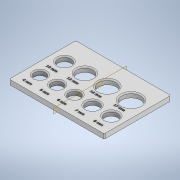
# Autodesk Inventor part: mmHexSocketSetOf9
Saved by Autodesk Inventor 2020.3 (Build 243373000, 373)
## iProperties
Created: 2020-03-13
Part Number: mmHexSocketSetOf9
Material: Generic
Document SubType Name: Modeling
Designer: robst
Density: 1 g/cm^3
Appearance: Default
Author: robst
Autodesk Inventor part; units mm, degrees
(part 1 of 2)
ref_plane "XZ Plane" through (0, 0, 0) normal (0, 1, 0) x (-1, 0, 0)
ref_plane "XY Plane" through (0, 0, 0) normal (0, 0, 1) x (1, 0, 0)
sketch "Sketch1" plane through (0, 0, 0) normal (0, 1, 0) x (-1, 0, 0)
  line L0 (63.5, 44.45) -> (-63.5, 44.45)
  line L1 (-63.5, 44.45) -> (-63.5, -44.45)
  line L2 (-63.5, -44.45) -> (63.5, -44.45)
  line L3 (63.5, -44.45) -> (63.5, 44.45)
  line L4 (63.5, 44.45) -> (-63.5, -44.45) construction
  line L5 (-63.5, 44.45) -> (63.5, -44.45) construction
  point P0 (0, 0)
  dimension "d3" = 88.9
  dimension "d13" = 127
  constraints: 12 end point, 2 midpoint, 2 parallel, 1 horizontal, 1 perpendicular
  measures "d3" distance of L2.end L0.start
  measures "d13" distance of L1.end L2.end
extrude "Extrusion1" add sketch "Sketch1" against normal blind 6.35
sketch "Sketch4" plane through (0, 0, 0) normal (0, 1, 0) x (1, 0, 0)
  line L0 (-63.5, -44.45) -> (-63.5, 44.45) construction
  line L1 (-63.5, -19.05) -> (63.5, -19.05) construction
  line L2 (63.5, 44.45) -> (63.5, -44.45) construction
  line L3 (-63.5, -44.45) -> (63.5, -44.45) projected
  circle A0 centre (-47.9975, -19.05) radius 7.62
  circle A1 centre (-24.8751, -19.05) radius 7.62
  circle A2 centre (-1.7526, -19.05) radius 7.62
  circle A3 centre (22.3859, -19.05) radius 8.636
  circle A4 centre (47.5403, -19.05) radius 8.636
  line L4 (-63.5, 12.7) -> (63.5, 12.7) construction
  circle A5 centre (-46.863, 12.7) radius 8.763
  circle A6 centre (-19.6215, 12.7) radius 10.6045
  circle A7 centre (10.414, 12.7) radius 11.557
  circle A8 centre (42.3545, 12.7) radius 12.5095
  point P0 (0, 0)
  dimension "d16" = 25.4
  dimension "hex4mmHole" = 15.24
  dimension "gap0" = 7.8825
  dimension "hex5mmHole" = 15.24
  dimension "gap1" = 23.1225
  dimension "hex6mmHole" = 15.24
  dimension "gap2" = 23.1225
  dimension "gap3" = 24.1385
  dimension "gap4" = 25.1545
  dimension "hex7mmHole" = 17.272
  dimension "hex8mmHole" = 17.272
  dimension "d27" = 7.3237
  dimension "frontToBackRowGap" = 31.75
  dimension "gap5" = 7.874
  dimension "hex10mmHole" = 17.526
  dimension "hex12mmHole" = 21.209
  dimension "gap6" = 27.2415
  dimension "hex14mmHole" = 23.114
  dimension "gap7" = 30.0355
  dimension "hex17mmHole" = 25.019
  dimension "gap8" = 31.9405
  dimension "d37" = 8.636
  constraints: 13 point on line, 9 centre point, 4 end point, 1 horizontal, 1 perpendicular
  measures "d16" distance between parallel lines of L1 L3
  measures "hex4mmHole" diameter of A0
  measures "gap0" distance edge to line of A0 L0
  measures "hex5mmHole" diameter of A1
  measures "gap1" distance of A1.centre A0.centre
  measures "hex6mmHole" diameter of A2
  measures "gap2" distance of A2.centre A1.centre
  measures "gap3" distance of A3.centre A2.centre
  measures "gap4" distance of A4.centre A3.centre
  measures "hex7mmHole" diameter of A3
  measures "hex8mmHole" diameter of A4
  measures "d27" distance edge to line of A4 L2
  measures "frontToBackRowGap" distance between parallel lines of L4 L1
  measures "gap5" distance edge to line of A5 L0
  measures "hex10mmHole" diameter of A5
  measures "hex12mmHole" diameter of A6
  measures "gap6" distance of A6.centre A5.centre
  measures "hex14mmHole" diameter of A7
  measures "gap7" distance of A7.centre A6.centre
  measures "hex17mmHole" diameter of A8
  measures "gap8" distance of A8.centre A7.centre
  measures "d37" distance edge to line of A8 L2
extrude "Extrusion3" cut sketch "Sketch4" against normal through all
sketch "Sketch7" plane through (0, 0, 0) normal (0, 1, 0) x (1, 0, 0)
  circle A0 centre (-47.9975, -19.05) radius 7.62 construction
  line L0 (63.5, -44.45) -> (-63.5, -44.45) construction
  line L1 (-55.6175, -35.6779) -> (-40.3775, -35.6779) construction
  line L2 (-32.4951, -35.6779) -> (-17.2551, -35.6779) construction
  line L3 (-9.3726, -35.6779) -> (5.8674, -35.6779) construction
  line L4 (13.7499, -35.6779) -> (30.7679, -35.6779) construction
  line L5 (38.6503, -35.6779) -> (55.6683, -35.6779) construction
  line L6 (-55.626, -3.81) -> (-38.354, -3.81) construction
  line L7 (-30.48, -3.81) -> (-7.62, -3.81) construction
  line L8 (0.254, -3.81) -> (23.114, -3.81) construction
  line L9 (30.988, -3.81) -> (55.626, -3.81) construction
  line L10 (-51.8572, -5.334) -> (-53.8702, -5.334)
  line L11 (-53.8702, -5.334) -> (-53.8702, -4.8029)
  line L12 (-53.8702, -4.8029) -> (-53.228, -4.8029)
  line L13 (-53.228, -4.8029) -> (-53.228, -3.19)
  line L14 (-53.228, -3.19) -> (-53.8702, -3.19)
  line L15 (-53.8702, -3.19) -> (-53.8702, -2.6936)
  spline S0 degree 2 poles (-53.8702, -2.6936) (-53.7294, -2.6936) (-53.4503, -2.6565) (-53.3663, -2.617) knots 0 0 0 1 2 2 2
  spline S1 degree 2 poles (-53.3663, -2.617) (-53.27, -2.5676) (-53.1613, -2.4021) (-53.1515, -2.2786) knots 0 0 0 1 2 2 2
  line L16 (-53.1515, -2.2786) -> (-52.4846, -2.2786)
  line L17 (-52.4846, -2.2786) -> (-52.4846, -4.8029)
  line L18 (-52.4846, -4.8029) -> (-51.8572, -4.8029)
  line L19 (-51.8572, -4.8029) -> (-51.8572, -5.334)
  spline S2 degree 2 poles (-49.0907, -3.81) (-49.0907, -4.2052) (-49.2167, -4.798) (-49.3575, -4.9981) knots 0 0 0 1 2 2 2
  spline S3 degree 2 poles (-49.3575, -4.9981) (-49.4958, -5.1957) (-49.9429, -5.3982) (-50.264, -5.3982) knots 0 0 0 1 2 2 2
  spline S4 degree 2 poles (-50.264, -5.3982) (-50.5876, -5.3982) (-51.0322, -5.1957) (-51.173, -4.9931) knots 0 0 0 1 2 2 2
  spline S5 degree 2 poles (-51.173, -4.9931) (-51.3138, -4.7931) (-51.4397, -4.2052) (-51.4397, -3.81) knots 0 0 0 1 2 2 2
  spline S6 degree 2 poles (-51.4397, -3.81) (-51.4397, -3.4049) (-51.3138, -2.8319) (-51.1705, -2.6244) knots 0 0 0 1 2 2 2
  spline S7 degree 2 poles (-51.1705, -2.6244) (-51.0272, -2.4219) (-50.5752, -2.2242) (-50.264, -2.2242) knots 0 0 0 1 2 2 2
  spline S8 degree 2 poles (-50.264, -2.2242) (-49.9355, -2.2242) (-49.4958, -2.4317) (-49.355, -2.6367) knots 0 0 0 1 2 2 2
  spline S9 degree 2 poles (-49.355, -2.6367) (-49.2167, -2.8368) (-49.0907, -3.4271) (-49.0907, -3.81) knots 0 0 0 1 2 2 2
  spline S10 degree 2 poles (-49.8589, -3.81) (-49.8589, -3.2444) (-50.0442, -2.7874) (-50.264, -2.7874) knots 0 0 0 1 2 2 2
  spline S11 degree 2 poles (-50.264, -2.7874) (-50.4838, -2.7874) (-50.6716, -3.2444) (-50.6716, -3.8125) knots 0 0 0 1 2 2 2
  spline S12 degree 2 poles (-50.6716, -3.8125) (-50.6716, -4.3707) (-50.4838, -4.8351) (-50.264, -4.8351) knots 0 0 0 1 2 2 2
  spline S13 degree 2 poles (-50.264, -4.8351) (-50.0466, -4.8351) (-49.8589, -4.3707) (-49.8589, -3.81) knots 0 0 0 1 2 2 2
  line L20 (-44.6842, -5.334) -> (-44.6842, -4.1854)
  spline S14 degree 2 poles (-44.6842, -4.1854) (-44.6842, -4.015) (-44.6966, -3.7828) (-44.7262, -3.7087) knots 0 0 0 1 2 2 2
  spline S15 degree 2 poles (-44.7262, -3.7087) (-44.7583, -3.6346) (-44.8868, -3.5679) (-45.0029, -3.5679) knots 0 0 0 1 2 2 2
  spline S16 degree 2 poles (-45.0029, -3.5679) (-45.0844, -3.5679) (-45.2425, -3.6396) (-45.3363, -3.7063) knots 0 0 0 1 2 2 2
  line L21 (-45.3363, -3.7063) -> (-45.3363, -5.334)
  line L22 (-45.3363, -5.334) -> (-46.0576, -5.334)
  line L23 (-46.0576, -5.334) -> (-46.0576, -4.1854)
  spline S17 degree 2 poles (-46.0576, -4.1854) (-46.0576, -4.0175) (-46.0724, -3.7828) (-46.102, -3.7087) knots 0 0 0 1 2 2 2
  spline S18 degree 2 poles (-46.102, -3.7087) (-46.1341, -3.6346) (-46.2626, -3.5679) (-46.3787, -3.5679) knots 0 0 0 1 2 2 2
  spline S19 degree 2 poles (-46.3787, -3.5679) (-46.4651, -3.5679) (-46.6356, -3.6494) (-46.7146, -3.7063) knots 0 0 0 1 2 2 2
  line L24 (-46.7146, -3.7063) -> (-46.7146, -5.334)
  line L25 (-46.7146, -5.334) -> (-47.4309, -5.334)
  line L26 (-47.4309, -5.334) -> (-47.4309, -3.0344)
  line L27 (-47.4309, -3.0344) -> (-46.7146, -3.0344)
  line L28 (-46.7146, -3.0344) -> (-46.7146, -3.2888)
  spline S20 degree 2 poles (-46.7146, -3.2888) (-46.5392, -3.1406) (-46.2255, -2.9727) (-46.0304, -2.9727) knots 0 0 0 1 2 2 2
  spline S21 degree 2 poles (-46.0304, -2.9727) (-45.8204, -2.9727) (-45.4993, -3.1727) (-45.4154, -3.3728) knots 0 0 0 1 2 2 2
  spline S22 degree 2 poles (-45.4154, -3.3728) (-45.2104, -3.1801) (-44.8448, -2.9727) (-44.6571, -2.9727) knots 0 0 0 1 2 2 2
  spline S23 degree 2 poles (-44.6571, -2.9727) (-44.4965, -2.9727) (-44.2421, -3.0739) (-44.1557, -3.1777) knots 0 0 0 1 2 2 2
  spline S24 degree 2 poles (-44.1557, -3.1777) (-44.0593, -3.2888) (-43.963, -3.5926) (-43.963, -3.8372) knots 0 0 0 1 2 2 2
  line L29 (-43.963, -3.8372) -> (-43.963, -5.334)
  line L30 (-43.963, -5.334) -> (-44.6842, -5.334)
  line L31 (-40.6878, -5.334) -> (-40.6878, -4.1854)
  spline S25 degree 2 poles (-40.6878, -4.1854) (-40.6878, -4.015) (-40.7001, -3.7828) (-40.7297, -3.7087) knots 0 0 0 1 2 2 2
  spline S26 degree 2 poles (-40.7297, -3.7087) (-40.7619, -3.6346) (-40.8903, -3.5679) (-41.0064, -3.5679) knots 0 0 0 1 2 2 2
  spline S27 degree 2 poles (-41.0064, -3.5679) (-41.0879, -3.5679) (-41.246, -3.6396) (-41.3398, -3.7063) knots 0 0 0 1 2 2 2
  line L32 (-41.3398, -3.7063) -> (-41.3398, -5.334)
  line L33 (-41.3398, -5.334) -> (-42.0611, -5.334)
  line L34 (-42.0611, -5.334) -> (-42.0611, -4.1854)
  spline S28 degree 2 poles (-42.0611, -4.1854) (-42.0611, -4.0175) (-42.0759, -3.7828) (-42.1055, -3.7087) knots 0 0 0 1 2 2 2
  spline S29 degree 2 poles (-42.1055, -3.7087) (-42.1377, -3.6346) (-42.2661, -3.5679) (-42.3822, -3.5679) knots 0 0 0 1 2 2 2
  spline S30 degree 2 poles (-42.3822, -3.5679) (-42.4686, -3.5679) (-42.6391, -3.6494) (-42.7181, -3.7063) knots 0 0 0 1 2 2 2
  line L35 (-42.7181, -3.7063) -> (-42.7181, -5.334)
  line L36 (-42.7181, -5.334) -> (-43.4344, -5.334)
  line L37 (-43.4344, -5.334) -> (-43.4344, -3.0344)
  line L38 (-43.4344, -3.0344) -> (-42.7181, -3.0344)
  line L39 (-42.7181, -3.0344) -> (-42.7181, -3.2888)
  spline S31 degree 2 poles (-42.7181, -3.2888) (-42.5427, -3.1406) (-42.229, -2.9727) (-42.0339, -2.9727) knots 0 0 0 1 2 2 2
  spline S32 degree 2 poles (-42.0339, -2.9727) (-41.824, -2.9727) (-41.5029, -3.1727) (-41.4189, -3.3728) knots 0 0 0 1 2 2 2
  spline S33 degree 2 poles (-41.4189, -3.3728) (-41.2139, -3.1801) (-40.8483, -2.9727) (-40.6606, -2.9727) knots 0 0 0 1 2 2 2
  spline S34 degree 2 poles (-40.6606, -2.9727) (-40.5, -2.9727) (-40.2456, -3.0739) (-40.1592, -3.1777) knots 0 0 0 1 2 2 2
  spline S35 degree 2 poles (-40.1592, -3.1777) (-40.0628, -3.2888) (-39.9665, -3.5926) (-39.9665, -3.8372) knots 0 0 0 1 2 2 2
  line L40 (-39.9665, -3.8372) -> (-39.9665, -5.334)
  line L41 (-39.9665, -5.334) -> (-40.6878, -5.334)
  line L42 (-23.9172, -5.334) -> (-25.9302, -5.334)
  line L43 (-25.9302, -5.334) -> (-25.9302, -4.8029)
  line L44 (-25.9302, -4.8029) -> (-25.288, -4.8029)
  line L45 (-25.288, -4.8029) -> (-25.288, -3.19)
  line L46 (-25.288, -3.19) -> (-25.9302, -3.19)
  line L47 (-25.9302, -3.19) -> (-25.9302, -2.6936)
  spline S36 degree 2 poles (-25.9302, -2.6936) (-25.7894, -2.6936) (-25.5103, -2.6565) (-25.4263, -2.617) knots 0 0 0 1 2 2 2
  spline S37 degree 2 poles (-25.4263, -2.617) (-25.33, -2.5676) (-25.2213, -2.4021) (-25.2115, -2.2786) knots 0 0 0 1 2 2 2
  line L48 (-25.2115, -2.2786) -> (-24.5446, -2.2786)
  line L49 (-24.5446, -2.2786) -> (-24.5446, -4.8029)
  line L50 (-24.5446, -4.8029) -> (-23.9172, -4.8029)
  line L51 (-23.9172, -4.8029) -> (-23.9172, -5.334)
  line L52 (-21.1112, -5.334) -> (-23.3515, -5.334)
  line L53 (-23.3515, -5.334) -> (-23.3515, -4.8375)
  spline S38 degree 2 poles (-23.3515, -4.8375) (-23.0675, -4.6103) (-22.613, -4.2101) (-22.4426, -4.0298) knots 0 0 0 1 2 2 2
  spline S39 degree 2 poles (-22.4426, -4.0298) (-22.2178, -3.7952) (-22.0177, -3.437) (-22.0177, -3.2493) knots 0 0 0 1 2 2 2
  spline S40 degree 2 poles (-22.0177, -3.2493) (-22.0177, -3.0369) (-22.2721, -2.8096) (-22.4994, -2.8096) knots 0 0 0 1 2 2 2
  spline S41 degree 2 poles (-22.4994, -2.8096) (-22.6155, -2.8096) (-22.8229, -2.8665) (-22.9292, -2.9109) knots 0 0 0 1 2 2 2
  spline S42 degree 2 poles (-22.9292, -2.9109) (-23.0329, -2.9578) (-23.1811, -3.0566) (-23.2182, -3.0813) knots 0 0 0 1 2 2 2
  line L54 (-23.2182, -3.0813) -> (-23.2774, -3.0813)
  line L55 (-23.2774, -3.0813) -> (-23.2774, -2.4169)
  spline S43 degree 2 poles (-23.2774, -2.4169) (-23.149, -2.3552) (-22.6006, -2.2267) (-22.3462, -2.2267) knots 0 0 0 1 2 2 2
  spline S44 degree 2 poles (-22.3462, -2.2267) (-21.8028, -2.2267) (-21.2446, -2.7108) (-21.2446, -3.148) knots 0 0 0 1 2 2 2
  spline S45 degree 2 poles (-21.2446, -3.148) (-21.2446, -3.4173) (-21.499, -3.936) (-21.793, -4.2324) knots 0 0 0 1 2 2 2
  spline S46 degree 2 poles (-21.793, -4.2324) (-21.9782, -4.4152) (-22.3265, -4.6992) (-22.403, -4.7585) knots 0 0 0 1 2 2 2
  line L56 (-22.403, -4.7585) -> (-21.1112, -4.7585)
  line L57 (-21.1112, -4.7585) -> (-21.1112, -5.334)
  line L58 (-16.7442, -5.334) -> (-16.7442, -4.1854)
  spline S47 degree 2 poles (-16.7442, -4.1854) (-16.7442, -4.015) (-16.7566, -3.7828) (-16.7862, -3.7087) knots 0 0 0 1 2 2 2
  spline S48 degree 2 poles (-16.7862, -3.7087) (-16.8183, -3.6346) (-16.9468, -3.5679) (-17.0629, -3.5679) knots 0 0 0 1 2 2 2
  spline S49 degree 2 poles (-17.0629, -3.5679) (-17.1444, -3.5679) (-17.3025, -3.6396) (-17.3963, -3.7063) knots 0 0 0 1 2 2 2
  line L59 (-17.3963, -3.7063) -> (-17.3963, -5.334)
  line L60 (-17.3963, -5.334) -> (-18.1176, -5.334)
  line L61 (-18.1176, -5.334) -> (-18.1176, -4.1854)
  spline S50 degree 2 poles (-18.1176, -4.1854) (-18.1176, -4.0175) (-18.1324, -3.7828) (-18.162, -3.7087) knots 0 0 0 1 2 2 2
  spline S51 degree 2 poles (-18.162, -3.7087) (-18.1941, -3.6346) (-18.3226, -3.5679) (-18.4387, -3.5679) knots 0 0 0 1 2 2 2
  spline S52 degree 2 poles (-18.4387, -3.5679) (-18.5251, -3.5679) (-18.6956, -3.6494) (-18.7746, -3.7063) knots 0 0 0 1 2 2 2
  line L62 (-18.7746, -3.7063) -> (-18.7746, -5.334)
  line L63 (-18.7746, -5.334) -> (-19.4909, -5.334)
  line L64 (-19.4909, -5.334) -> (-19.4909, -3.0344)
  line L65 (-19.4909, -3.0344) -> (-18.7746, -3.0344)
  line L66 (-18.7746, -3.0344) -> (-18.7746, -3.2888)
  spline S53 degree 2 poles (-18.7746, -3.2888) (-18.5992, -3.1406) (-18.2855, -2.9727) (-18.0904, -2.9727) knots 0 0 0 1 2 2 2
  spline S54 degree 2 poles (-18.0904, -2.9727) (-17.8804, -2.9727) (-17.5593, -3.1727) (-17.4754, -3.3728) knots 0 0 0 1 2 2 2
  spline S55 degree 2 poles (-17.4754, -3.3728) (-17.2704, -3.1801) (-16.9048, -2.9727) (-16.7171, -2.9727) knots 0 0 0 1 2 2 2
  spline S56 degree 2 poles (-16.7171, -2.9727) (-16.5565, -2.9727) (-16.3021, -3.0739) (-16.2157, -3.1777) knots 0 0 0 1 2 2 2
  spline S57 degree 2 poles (-16.2157, -3.1777) (-16.1193, -3.2888) (-16.023, -3.5926) (-16.023, -3.8372) knots 0 0 0 1 2 2 2
  line L67 (-16.023, -3.8372) -> (-16.023, -5.334)
  line L68 (-16.023, -5.334) -> (-16.7442, -5.334)
  line L69 (-12.7478, -5.334) -> (-12.7478, -4.1854)
  spline S58 degree 2 poles (-12.7478, -4.1854) (-12.7478, -4.015) (-12.7601, -3.7828) (-12.7897, -3.7087) knots 0 0 0 1 2 2 2
  spline S59 degree 2 poles (-12.7897, -3.7087) (-12.8219, -3.6346) (-12.9503, -3.5679) (-13.0664, -3.5679) knots 0 0 0 1 2 2 2
  spline S60 degree 2 poles (-13.0664, -3.5679) (-13.1479, -3.5679) (-13.306, -3.6396) (-13.3998, -3.7063) knots 0 0 0 1 2 2 2
  line L70 (-13.3998, -3.7063) -> (-13.3998, -5.334)
  line L71 (-13.3998, -5.334) -> (-14.1211, -5.334)
  line L72 (-14.1211, -5.334) -> (-14.1211, -4.1854)
  spline S61 degree 2 poles (-14.1211, -4.1854) (-14.1211, -4.0175) (-14.1359, -3.7828) (-14.1655, -3.7087) knots 0 0 0 1 2 2 2
  spline S62 degree 2 poles (-14.1655, -3.7087) (-14.1977, -3.6346) (-14.3261, -3.5679) (-14.4422, -3.5679) knots 0 0 0 1 2 2 2
  spline S63 degree 2 poles (-14.4422, -3.5679) (-14.5286, -3.5679) (-14.6991, -3.6494) (-14.7781, -3.7063) knots 0 0 0 1 2 2 2
  line L73 (-14.7781, -3.7063) -> (-14.7781, -5.334)
  line L74 (-14.7781, -5.334) -> (-15.4944, -5.334)
  line L75 (-15.4944, -5.334) -> (-15.4944, -3.0344)
  line L76 (-15.4944, -3.0344) -> (-14.7781, -3.0344)
  line L77 (-14.7781, -3.0344) -> (-14.7781, -3.2888)
  spline S64 degree 2 poles (-14.7781, -3.2888) (-14.6027, -3.1406) (-14.289, -2.9727) (-14.0939, -2.9727) knots 0 0 0 1 2 2 2
  spline S65 degree 2 poles (-14.0939, -2.9727) (-13.884, -2.9727) (-13.5629, -3.1727) (-13.4789, -3.3728) knots 0 0 0 1 2 2 2
  spline S66 degree 2 poles (-13.4789, -3.3728) (-13.2739, -3.1801) (-12.9083, -2.9727) (-12.7206, -2.9727) knots 0 0 0 1 2 2 2
  spline S67 degree 2 poles (-12.7206, -2.9727) (-12.56, -2.9727) (-12.3056, -3.0739) (-12.2192, -3.1777) knots 0 0 0 1 2 2 2
  spline S68 degree 2 poles (-12.2192, -3.1777) (-12.1228, -3.2888) (-12.0265, -3.5926) (-12.0265, -3.8372) knots 0 0 0 1 2 2 2
  line L78 (-12.0265, -3.8372) -> (-12.0265, -5.334)
  line L79 (-12.0265, -5.334) -> (-12.7478, -5.334)
  line L80 (6.8168, -5.334) -> (4.8038, -5.334)
  line L81 (4.8038, -5.334) -> (4.8038, -4.8029)
  line L82 (4.8038, -4.8029) -> (5.446, -4.8029)
  line L83 (5.446, -4.8029) -> (5.446, -3.19)
  line L84 (5.446, -3.19) -> (4.8038, -3.19)
  line L85 (4.8038, -3.19) -> (4.8038, -2.6936)
  spline S69 degree 2 poles (4.8038, -2.6936) (4.9446, -2.6936) (5.2237, -2.6565) (5.3077, -2.617) knots 0 0 0 1 2 2 2
  spline S70 degree 2 poles (5.3077, -2.617) (5.404, -2.5676) (5.5127, -2.4021) (5.5225, -2.2786) knots 0 0 0 1 2 2 2
  line L86 (5.5225, -2.2786) -> (6.1894, -2.2786)
  line L87 (6.1894, -2.2786) -> (6.1894, -4.8029)
  line L88 (6.1894, -4.8029) -> (6.8168, -4.8029)
  line L89 (6.8168, -4.8029) -> (6.8168, -5.334)
  line L90 (9.6598, -4.6226) -> (9.2473, -4.6226)
  line L91 (9.2473, -4.6226) -> (9.2473, -5.3414)
  line L92 (9.2473, -5.3414) -> (8.5088, -5.3414)
  line L93 (8.5088, -5.3414) -> (8.5088, -4.6226)
  line L94 (8.5088, -4.6226) -> (7.1651, -4.6226)
  line L95 (7.1651, -4.6226) -> (7.1651, -4.0545)
  line L96 (7.1651, -4.0545) -> (8.4841, -2.286)
  line L97 (8.4841, -2.286) -> (9.2473, -2.286)
  line L98 (9.2473, -2.286) -> (9.2473, -4.0743)
  line L99 (9.2473, -4.0743) -> (9.6598, -4.0743)
  line L100 (9.6598, -4.0743) -> (9.6598, -4.6226)
  line L101 (8.5088, -4.0743) -> (8.5088, -3.0369)
  line L102 (8.5088, -3.0369) -> (7.7357, -4.0743)
  line L103 (7.7357, -4.0743) -> (8.5088, -4.0743)
  line L104 (13.9898, -5.334) -> (13.9898, -4.1854)
  spline S71 degree 2 poles (13.9898, -4.1854) (13.9898, -4.015) (13.9774, -3.7828) (13.9478, -3.7087) knots 0 0 0 1 2 2 2
  spline S72 degree 2 poles (13.9478, -3.7087) (13.9157, -3.6346) (13.7872, -3.5679) (13.6711, -3.5679) knots 0 0 0 1 2 2 2
  spline S73 degree 2 poles (13.6711, -3.5679) (13.5896, -3.5679) (13.4315, -3.6396) (13.3377, -3.7063) knots 0 0 0 1 2 2 2
  line L105 (13.3377, -3.7063) -> (13.3377, -5.334)
  line L106 (13.3377, -5.334) -> (12.6164, -5.334)
  line L107 (12.6164, -5.334) -> (12.6164, -4.1854)
  spline S74 degree 2 poles (12.6164, -4.1854) (12.6164, -4.0175) (12.6016, -3.7828) (12.572, -3.7087) knots 0 0 0 1 2 2 2
  spline S75 degree 2 poles (12.572, -3.7087) (12.5399, -3.6346) (12.4114, -3.5679) (12.2953, -3.5679) knots 0 0 0 1 2 2 2
  spline S76 degree 2 poles (12.2953, -3.5679) (12.2089, -3.5679) (12.0384, -3.6494) (11.9594, -3.7063) knots 0 0 0 1 2 2 2
  line L108 (11.9594, -3.7063) -> (11.9594, -5.334)
  line L109 (11.9594, -5.334) -> (11.2431, -5.334)
  line L110 (11.2431, -5.334) -> (11.2431, -3.0344)
  line L111 (11.2431, -3.0344) -> (11.9594, -3.0344)
  line L112 (11.9594, -3.0344) -> (11.9594, -3.2888)
  spline S77 degree 2 poles (11.9594, -3.2888) (12.1348, -3.1406) (12.4485, -2.9727) (12.6436, -2.9727) knots 0 0 0 1 2 2 2
  spline S78 degree 2 poles (12.6436, -2.9727) (12.8536, -2.9727) (13.1747, -3.1727) (13.2586, -3.3728) knots 0 0 0 1 2 2 2
  spline S79 degree 2 poles (13.2586, -3.3728) (13.4636, -3.1801) (13.8292, -2.9727) (14.0169, -2.9727) knots 0 0 0 1 2 2 2
  spline S80 degree 2 poles (14.0169, -2.9727) (14.1775, -2.9727) (14.4319, -3.0739) (14.5183, -3.1777) knots 0 0 0 1 2 2 2
  spline S81 degree 2 poles (14.5183, -3.1777) (14.6147, -3.2888) (14.711, -3.5926) (14.711, -3.8372) knots 0 0 0 1 2 2 2
  line L113 (14.711, -3.8372) -> (14.711, -5.334)
  line L114 (14.711, -5.334) -> (13.9898, -5.334)
  line L115 (17.9862, -5.334) -> (17.9862, -4.1854)
  spline S82 degree 2 poles (17.9862, -4.1854) (17.9862, -4.015) (17.9739, -3.7828) (17.9443, -3.7087) knots 0 0 0 1 2 2 2
  spline S83 degree 2 poles (17.9443, -3.7087) (17.9121, -3.6346) (17.7837, -3.5679) (17.6676, -3.5679) knots 0 0 0 1 2 2 2
  spline S84 degree 2 poles (17.6676, -3.5679) (17.5861, -3.5679) (17.428, -3.6396) (17.3342, -3.7063) knots 0 0 0 1 2 2 2
  line L116 (17.3342, -3.7063) -> (17.3342, -5.334)
  line L117 (17.3342, -5.334) -> (16.6129, -5.334)
  line L118 (16.6129, -5.334) -> (16.6129, -4.1854)
  spline S85 degree 2 poles (16.6129, -4.1854) (16.6129, -4.0175) (16.5981, -3.7828) (16.5685, -3.7087) knots 0 0 0 1 2 2 2
  spline S86 degree 2 poles (16.5685, -3.7087) (16.5363, -3.6346) (16.4079, -3.5679) (16.2918, -3.5679) knots 0 0 0 1 2 2 2
  spline S87 degree 2 poles (16.2918, -3.5679) (16.2054, -3.5679) (16.0349, -3.6494) (15.9559, -3.7063) knots 0 0 0 1 2 2 2
  line L119 (15.9559, -3.7063) -> (15.9559, -5.334)
  line L120 (15.9559, -5.334) -> (15.2396, -5.334)
  line L121 (15.2396, -5.334) -> (15.2396, -3.0344)
  line L122 (15.2396, -3.0344) -> (15.9559, -3.0344)
  line L123 (15.9559, -3.0344) -> (15.9559, -3.2888)
  spline S88 degree 2 poles (15.9559, -3.2888) (16.1313, -3.1406) (16.445, -2.9727) (16.6401, -2.9727) knots 0 0 0 1 2 2 2
  spline S89 degree 2 poles (16.6401, -2.9727) (16.85, -2.9727) (17.1711, -3.1727) (17.2551, -3.3728) knots 0 0 0 1 2 2 2
  spline S90 degree 2 poles (17.2551, -3.3728) (17.4601, -3.1801) (17.8257, -2.9727) (18.0134, -2.9727) knots 0 0 0 1 2 2 2
  spline S91 degree 2 poles (18.0134, -2.9727) (18.174, -2.9727) (18.4284, -3.0739) (18.5148, -3.1777) knots 0 0 0 1 2 2 2
  spline S92 degree 2 poles (18.5148, -3.1777) (18.6112, -3.2888) (18.7075, -3.5926) (18.7075, -3.8372) knots 0 0 0 1 2 2 2
  line L124 (18.7075, -3.8372) -> (18.7075, -5.334)
  line L125 (18.7075, -5.334) -> (17.9862, -5.334)
  line L126 (38.4398, -5.334) -> (36.4268, -5.334)
  line L127 (36.4268, -5.334) -> (36.4268, -4.8029)
  line L128 (36.4268, -4.8029) -> (37.069, -4.8029)
  line L129 (37.069, -4.8029) -> (37.069, -3.19)
  line L130 (37.069, -3.19) -> (36.4268, -3.19)
  line L131 (36.4268, -3.19) -> (36.4268, -2.6936)
  spline S93 degree 2 poles (36.4268, -2.6936) (36.5676, -2.6936) (36.8467, -2.6565) (36.9307, -2.617) knots 0 0 0 1 2 2 2
  spline S94 degree 2 poles (36.9307, -2.617) (37.027, -2.5676) (37.1357, -2.4021) (37.1455, -2.2786) knots 0 0 0 1 2 2 2
  line L132 (37.1455, -2.2786) -> (37.8124, -2.2786)
  line L133 (37.8124, -2.2786) -> (37.8124, -4.8029)
  line L134 (37.8124, -4.8029) -> (38.4398, -4.8029)
  line L135 (38.4398, -4.8029) -> (38.4398, -5.334)
  line L136 (41.1791, -2.8912) -> (39.8774, -5.334)
  line L137 (39.8774, -5.334) -> (39.0277, -5.334)
  line L138 (39.0277, -5.334) -> (40.3887, -2.8615)
  line L139 (40.3887, -2.8615) -> (38.9363, -2.8615)
  line L140 (38.9363, -2.8615) -> (38.9363, -2.286)
  line L141 (38.9363, -2.286) -> (41.1791, -2.286)
  line L142 (41.1791, -2.286) -> (41.1791, -2.8912)
  line L143 (45.6128, -5.334) -> (45.6128, -4.1854)
  spline S95 degree 2 poles (45.6128, -4.1854) (45.6128, -4.015) (45.6004, -3.7828) (45.5708, -3.7087) knots 0 0 0 1 2 2 2
  spline S96 degree 2 poles (45.5708, -3.7087) (45.5387, -3.6346) (45.4102, -3.5679) (45.2941, -3.5679) knots 0 0 0 1 2 2 2
  spline S97 degree 2 poles (45.2941, -3.5679) (45.2126, -3.5679) (45.0545, -3.6396) (44.9607, -3.7063) knots 0 0 0 1 2 2 2
  line L144 (44.9607, -3.7063) -> (44.9607, -5.334)
  line L145 (44.9607, -5.334) -> (44.2394, -5.334)
  line L146 (44.2394, -5.334) -> (44.2394, -4.1854)
  spline S98 degree 2 poles (44.2394, -4.1854) (44.2394, -4.0175) (44.2246, -3.7828) (44.195, -3.7087) knots 0 0 0 1 2 2 2
  spline S99 degree 2 poles (44.195, -3.7087) (44.1629, -3.6346) (44.0344, -3.5679) (43.9183, -3.5679) knots 0 0 0 1 2 2 2
  spline S100 degree 2 poles (43.9183, -3.5679) (43.8319, -3.5679) (43.6614, -3.6494) (43.5824, -3.7063) knots 0 0 0 1 2 2 2
  line L147 (43.5824, -3.7063) -> (43.5824, -5.334)
  line L148 (43.5824, -5.334) -> (42.8661, -5.334)
  line L149 (42.8661, -5.334) -> (42.8661, -3.0344)
  line L150 (42.8661, -3.0344) -> (43.5824, -3.0344)
  line L151 (43.5824, -3.0344) -> (43.5824, -3.2888)
  spline S101 degree 2 poles (43.5824, -3.2888) (43.7578, -3.1406) (44.0715, -2.9727) (44.2666, -2.9727) knots 0 0 0 1 2 2 2
  spline S102 degree 2 poles (44.2666, -2.9727) (44.4766, -2.9727) (44.7977, -3.1727) (44.8816, -3.3728) knots 0 0 0 1 2 2 2
  spline S103 degree 2 poles (44.8816, -3.3728) (45.0866, -3.1801) (45.4522, -2.9727) (45.6399, -2.9727) knots 0 0 0 1 2 2 2
  spline S104 degree 2 poles (45.6399, -2.9727) (45.8005, -2.9727) (46.0549, -3.0739) (46.1413, -3.1777) knots 0 0 0 1 2 2 2
  spline S105 degree 2 poles (46.1413, -3.1777) (46.2377, -3.2888) (46.334, -3.5926) (46.334, -3.8372) knots 0 0 0 1 2 2 2
  line L152 (46.334, -3.8372) -> (46.334, -5.334)
  line L153 (46.334, -5.334) -> (45.6128, -5.334)
  line L154 (49.6092, -5.334) -> (49.6092, -4.1854)
  spline S106 degree 2 poles (49.6092, -4.1854) (49.6092, -4.015) (49.5969, -3.7828) (49.5673, -3.7087) knots 0 0 0 1 2 2 2
  spline S107 degree 2 poles (49.5673, -3.7087) (49.5351, -3.6346) (49.4067, -3.5679) (49.2906, -3.5679) knots 0 0 0 1 2 2 2
  spline S108 degree 2 poles (49.2906, -3.5679) (49.2091, -3.5679) (49.051, -3.6396) (48.9572, -3.7063) knots 0 0 0 1 2 2 2
  line L155 (48.9572, -3.7063) -> (48.9572, -5.334)
  line L156 (48.9572, -5.334) -> (48.2359, -5.334)
  line L157 (48.2359, -5.334) -> (48.2359, -4.1854)
  spline S109 degree 2 poles (48.2359, -4.1854) (48.2359, -4.0175) (48.2211, -3.7828) (48.1915, -3.7087) knots 0 0 0 1 2 2 2
  spline S110 degree 2 poles (48.1915, -3.7087) (48.1593, -3.6346) (48.0309, -3.5679) (47.9148, -3.5679) knots 0 0 0 1 2 2 2
  spline S111 degree 2 poles (47.9148, -3.5679) (47.8284, -3.5679) (47.6579, -3.6494) (47.5789, -3.7063) knots 0 0 0 1 2 2 2
  line L158 (47.5789, -3.7063) -> (47.5789, -5.334)
  line L159 (47.5789, -5.334) -> (46.8626, -5.334)
  line L160 (46.8626, -5.334) -> (46.8626, -3.0344)
  line L161 (46.8626, -3.0344) -> (47.5789, -3.0344)
  line L162 (47.5789, -3.0344) -> (47.5789, -3.2888)
  spline S112 degree 2 poles (47.5789, -3.2888) (47.7543, -3.1406) (48.068, -2.9727) (48.2631, -2.9727) knots 0 0 0 1 2 2 2
  spline S113 degree 2 poles (48.2631, -2.9727) (48.473, -2.9727) (48.7941, -3.1727) (48.8781, -3.3728) knots 0 0 0 1 2 2 2
  spline S114 degree 2 poles (48.8781, -3.3728) (49.0831, -3.1801) (49.4487, -2.9727) (49.6364, -2.9727) knots 0 0 0 1 2 2 2
  spline S115 degree 2 poles (49.6364, -2.9727) (49.797, -2.9727) (50.0514, -3.0739) (50.1378, -3.1777) knots 0 0 0 1 2 2 2
  spline S116 degree 2 poles (50.1378, -3.1777) (50.2342, -3.2888) (50.3305, -3.5926) (50.3305, -3.8372) knots 0 0 0 1 2 2 2
  line L163 (50.3305, -3.8372) -> (50.3305, -5.334)
  line L164 (50.3305, -5.334) -> (49.6092, -5.334)
  line L165 (-51.3568, -36.4905) -> (-51.7692, -36.4905)
  line L166 (-51.7692, -36.4905) -> (-51.7692, -37.2093)
  line L167 (-51.7692, -37.2093) -> (-52.5078, -37.2093)
  line L168 (-52.5078, -37.2093) -> (-52.5078, -36.4905)
  line L169 (-52.5078, -36.4905) -> (-53.8515, -36.4905)
  line L170 (-53.8515, -36.4905) -> (-53.8515, -35.9224)
  line L171 (-53.8515, -35.9224) -> (-52.5325, -34.1539)
  line L172 (-52.5325, -34.1539) -> (-51.7692, -34.1539)
  line L173 (-51.7692, -34.1539) -> (-51.7692, -35.9422)
  line L174 (-51.7692, -35.9422) -> (-51.3568, -35.9422)
  line L175 (-51.3568, -35.9422) -> (-51.3568, -36.4905)
  line L176 (-52.5078, -35.9422) -> (-52.5078, -34.9048)
  line L177 (-52.5078, -34.9048) -> (-53.2809, -35.9422)
  line L178 (-53.2809, -35.9422) -> (-52.5078, -35.9422)
  line L179 (-47.0268, -37.2019) -> (-47.0268, -36.0533)
  spline S117 degree 2 poles (-47.0268, -36.0533) (-47.0268, -35.8829) (-47.0392, -35.6507) (-47.0688, -35.5766) knots 0 0 0 1 2 2 2
  spline S118 degree 2 poles (-47.0688, -35.5766) (-47.1009, -35.5025) (-47.2294, -35.4358) (-47.3454, -35.4358) knots 0 0 0 1 2 2 2
  spline S119 degree 2 poles (-47.3454, -35.4358) (-47.427, -35.4358) (-47.585, -35.5074) (-47.6789, -35.5741) knots 0 0 0 1 2 2 2
  line L180 (-47.6789, -35.5741) -> (-47.6789, -37.2019)
  line L181 (-47.6789, -37.2019) -> (-48.4001, -37.2019)
  line L182 (-48.4001, -37.2019) -> (-48.4001, -36.0533)
  spline S120 degree 2 poles (-48.4001, -36.0533) (-48.4001, -35.8853) (-48.415, -35.6507) (-48.4446, -35.5766) knots 0 0 0 1 2 2 2
  spline S121 degree 2 poles (-48.4446, -35.5766) (-48.4767, -35.5025) (-48.6052, -35.4358) (-48.7212, -35.4358) knots 0 0 0 1 2 2 2
  spline S122 degree 2 poles (-48.7212, -35.4358) (-48.8077, -35.4358) (-48.9781, -35.5173) (-49.0572, -35.5741) knots 0 0 0 1 2 2 2
  line L183 (-49.0572, -35.5741) -> (-49.0572, -37.2019)
  line L184 (-49.0572, -37.2019) -> (-49.7735, -37.2019)
  line L185 (-49.7735, -37.2019) -> (-49.7735, -34.9023)
  line L186 (-49.7735, -34.9023) -> (-49.0572, -34.9023)
  line L187 (-49.0572, -34.9023) -> (-49.0572, -35.1567)
  spline S123 degree 2 poles (-49.0572, -35.1567) (-48.8818, -35.0085) (-48.5681, -34.8405) (-48.373, -34.8405) knots 0 0 0 1 2 2 2
  spline S124 degree 2 poles (-48.373, -34.8405) (-48.163, -34.8405) (-47.8419, -35.0406) (-47.7579, -35.2407) knots 0 0 0 1 2 2 2
  spline S125 degree 2 poles (-47.7579, -35.2407) (-47.5529, -35.048) (-47.1874, -34.8405) (-46.9996, -34.8405) knots 0 0 0 1 2 2 2
  spline S126 degree 2 poles (-46.9996, -34.8405) (-46.8391, -34.8405) (-46.5847, -34.9418) (-46.4982, -35.0455) knots 0 0 0 1 2 2 2
  spline S127 degree 2 poles (-46.4982, -35.0455) (-46.4019, -35.1567) (-46.3056, -35.4605) (-46.3056, -35.705) knots 0 0 0 1 2 2 2
  line L188 (-46.3056, -35.705) -> (-46.3056, -37.2019)
  line L189 (-46.3056, -37.2019) -> (-47.0268, -37.2019)
  line L190 (-43.0303, -37.2019) -> (-43.0303, -36.0533)
  spline S128 degree 2 poles (-43.0303, -36.0533) (-43.0303, -35.8829) (-43.0427, -35.6507) (-43.0723, -35.5766) knots 0 0 0 1 2 2 2
  spline S129 degree 2 poles (-43.0723, -35.5766) (-43.1044, -35.5025) (-43.2329, -35.4358) (-43.349, -35.4358) knots 0 0 0 1 2 2 2
  spline S130 degree 2 poles (-43.349, -35.4358) (-43.4305, -35.4358) (-43.5886, -35.5074) (-43.6824, -35.5741) knots 0 0 0 1 2 2 2
  line L191 (-43.6824, -35.5741) -> (-43.6824, -37.2019)
  line L192 (-43.6824, -37.2019) -> (-44.4037, -37.2019)
  line L193 (-44.4037, -37.2019) -> (-44.4037, -36.0533)
  spline S131 degree 2 poles (-44.4037, -36.0533) (-44.4037, -35.8853) (-44.4185, -35.6507) (-44.4481, -35.5766) knots 0 0 0 1 2 2 2
  spline S132 degree 2 poles (-44.4481, -35.5766) (-44.4802, -35.5025) (-44.6087, -35.4358) (-44.7248, -35.4358) knots 0 0 0 1 2 2 2
  spline S133 degree 2 poles (-44.7248, -35.4358) (-44.8112, -35.4358) (-44.9816, -35.5173) (-45.0607, -35.5741) knots 0 0 0 1 2 2 2
  line L194 (-45.0607, -35.5741) -> (-45.0607, -37.2019)
  line L195 (-45.0607, -37.2019) -> (-45.777, -37.2019)
  line L196 (-45.777, -37.2019) -> (-45.777, -34.9023)
  line L197 (-45.777, -34.9023) -> (-45.0607, -34.9023)
  line L198 (-45.0607, -34.9023) -> (-45.0607, -35.1567)
  spline S134 degree 2 poles (-45.0607, -35.1567) (-44.8853, -35.0085) (-44.5716, -34.8405) (-44.3765, -34.8405) knots 0 0 0 1 2 2 2
  spline S135 degree 2 poles (-44.3765, -34.8405) (-44.1665, -34.8405) (-43.8454, -35.0406) (-43.7615, -35.2407) knots 0 0 0 1 2 2 2
  spline S136 degree 2 poles (-43.7615, -35.2407) (-43.5564, -35.048) (-43.1909, -34.8405) (-43.0032, -34.8405) knots 0 0 0 1 2 2 2
  spline S137 degree 2 poles (-43.0032, -34.8405) (-42.8426, -34.8405) (-42.5882, -34.9418) (-42.5017, -35.0455) knots 0 0 0 1 2 2 2
  spline S138 degree 2 poles (-42.5017, -35.0455) (-42.4054, -35.1567) (-42.3091, -35.4605) (-42.3091, -35.705) knots 0 0 0 1 2 2 2
  line L199 (-42.3091, -35.705) -> (-42.3091, -37.2019)
  line L200 (-42.3091, -37.2019) -> (-43.0303, -37.2019)
  spline S139 degree 2 poles (-28.3405, -36.1694) (-28.3405, -36.409) (-28.5035, -36.8141) (-28.6641, -36.9598) knots 0 0 0 1 2 2 2
  spline S140 degree 2 poles (-28.6641, -36.9598) (-28.8246, -37.1055) (-29.2643, -37.2661) (-29.5854, -37.2661) knots 0 0 0 1 2 2 2
  spline S141 degree 2 poles (-29.5854, -37.2661) (-29.9262, -37.2636) (-30.4153, -37.1525) (-30.5759, -37.0808) knots 0 0 0 1 2 2 2
  line L201 (-30.5759, -37.0808) -> (-30.5759, -36.4164)
  line L202 (-30.5759, -36.4164) -> (-30.5067, -36.4164)
  spline S142 degree 2 poles (-30.5067, -36.4164) (-30.4474, -36.4485) (-30.3042, -36.5325) (-30.1881, -36.577) knots 0 0 0 1 2 2 2
  spline S143 degree 2 poles (-30.1881, -36.577) (-30.0794, -36.6189) (-29.8546, -36.6758) (-29.7188, -36.6758) knots 0 0 0 1 2 2 2
  spline S144 degree 2 poles (-29.7188, -36.6758) (-29.6002, -36.6758) (-29.3236, -36.6165) (-29.2396, -36.5374) knots 0 0 0 1 2 2 2
  spline S145 degree 2 poles (-29.2396, -36.5374) (-29.1778, -36.4757) (-29.1087, -36.325) (-29.1087, -36.199) knots 0 0 0 1 2 2 2
  spline S146 degree 2 poles (-29.1087, -36.199) (-29.1087, -36.0904) (-29.1976, -35.9372) (-29.2692, -35.8903) knots 0 0 0 1 2 2 2
  spline S147 degree 2 poles (-29.2692, -35.8903) (-29.373, -35.8211) (-29.6694, -35.7816) (-29.7756, -35.7816) knots 0 0 0 1 2 2 2
  spline S148 degree 2 poles (-29.7756, -35.7816) (-29.9435, -35.7816) (-30.2622, -35.8359) (-30.3783, -35.8656) knots 0 0 0 1 2 2 2
  line L203 (-30.3783, -35.8656) -> (-30.445, -35.8656)
  line L204 (-30.445, -35.8656) -> (-30.445, -34.1539)
  line L205 (-30.445, -34.1539) -> (-28.4245, -34.1539)
  line L206 (-28.4245, -34.1539) -> (-28.4245, -34.7294)
  line L207 (-28.4245, -34.7294) -> (-29.7212, -34.7294)
  line L208 (-29.7212, -34.7294) -> (-29.7212, -35.2357)
  spline S149 degree 2 poles (-29.7212, -35.2357) (-29.6595, -35.2308) (-29.4891, -35.2259) (-29.4421, -35.2259) knots 0 0 0 1 2 2 2
  spline S150 degree 2 poles (-29.4421, -35.2259) (-29.2223, -35.2259) (-28.8518, -35.3148) (-28.7061, -35.4062) knots 0 0 0 1 2 2 2
  spline S151 degree 2 poles (-28.7061, -35.4062) (-28.5332, -35.5198) (-28.3405, -35.8977) (-28.3405, -36.1694) knots 0 0 0 1 2 2 2
  line L209 (-23.9044, -37.2019) -> (-23.9044, -36.0533)
  spline S152 degree 2 poles (-23.9044, -36.0533) (-23.9044, -35.8829) (-23.9167, -35.6507) (-23.9463, -35.5766) knots 0 0 0 1 2 2 2
  spline S153 degree 2 poles (-23.9463, -35.5766) (-23.9785, -35.5025) (-24.1069, -35.4358) (-24.223, -35.4358) knots 0 0 0 1 2 2 2
  spline S154 degree 2 poles (-24.223, -35.4358) (-24.3045, -35.4358) (-24.4626, -35.5074) (-24.5564, -35.5741) knots 0 0 0 1 2 2 2
  line L210 (-24.5564, -35.5741) -> (-24.5564, -37.2019)
  line L211 (-24.5564, -37.2019) -> (-25.2777, -37.2019)
  line L212 (-25.2777, -37.2019) -> (-25.2777, -36.0533)
  spline S155 degree 2 poles (-25.2777, -36.0533) (-25.2777, -35.8853) (-25.2925, -35.6507) (-25.3221, -35.5766) knots 0 0 0 1 2 2 2
  spline S156 degree 2 poles (-25.3221, -35.5766) (-25.3542, -35.5025) (-25.4827, -35.4358) (-25.5988, -35.4358) knots 0 0 0 1 2 2 2
  spline S157 degree 2 poles (-25.5988, -35.4358) (-25.6852, -35.4358) (-25.8557, -35.5173) (-25.9347, -35.5741) knots 0 0 0 1 2 2 2
  line L213 (-25.9347, -35.5741) -> (-25.9347, -37.2019)
  line L214 (-25.9347, -37.2019) -> (-26.651, -37.2019)
  line L215 (-26.651, -37.2019) -> (-26.651, -34.9023)
  line L216 (-26.651, -34.9023) -> (-25.9347, -34.9023)
  line L217 (-25.9347, -34.9023) -> (-25.9347, -35.1567)
  spline S158 degree 2 poles (-25.9347, -35.1567) (-25.7593, -35.0085) (-25.4456, -34.8405) (-25.2505, -34.8405) knots 0 0 0 1 2 2 2
  spline S159 degree 2 poles (-25.2505, -34.8405) (-25.0406, -34.8405) (-24.7195, -35.0406) (-24.6355, -35.2407) knots 0 0 0 1 2 2 2
  spline S160 degree 2 poles (-24.6355, -35.2407) (-24.4305, -35.048) (-24.0649, -34.8405) (-23.8772, -34.8405) knots 0 0 0 1 2 2 2
  spline S161 degree 2 poles (-23.8772, -34.8405) (-23.7166, -34.8405) (-23.4622, -34.9418) (-23.3758, -35.0455) knots 0 0 0 1 2 2 2
  spline S162 degree 2 poles (-23.3758, -35.0455) (-23.2794, -35.1567) (-23.1831, -35.4605) (-23.1831, -35.705) knots 0 0 0 1 2 2 2
  line L218 (-23.1831, -35.705) -> (-23.1831, -37.2019)
  line L219 (-23.1831, -37.2019) -> (-23.9044, -37.2019)
  line L220 (-19.9079, -37.2019) -> (-19.9079, -36.0533)
  spline S163 degree 2 poles (-19.9079, -36.0533) (-19.9079, -35.8829) (-19.9202, -35.6507) (-19.9499, -35.5766) knots 0 0 0 1 2 2 2
  spline S164 degree 2 poles (-19.9499, -35.5766) (-19.982, -35.5025) (-20.1104, -35.4358) (-20.2265, -35.4358) knots 0 0 0 1 2 2 2
  spline S165 degree 2 poles (-20.2265, -35.4358) (-20.308, -35.4358) (-20.4661, -35.5074) (-20.5599, -35.5741) knots 0 0 0 1 2 2 2
  line L221 (-20.5599, -35.5741) -> (-20.5599, -37.2019)
  line L222 (-20.5599, -37.2019) -> (-21.2812, -37.2019)
  line L223 (-21.2812, -37.2019) -> (-21.2812, -36.0533)
  spline S166 degree 2 poles (-21.2812, -36.0533) (-21.2812, -35.8853) (-21.296, -35.6507) (-21.3257, -35.5766) knots 0 0 0 1 2 2 2
  spline S167 degree 2 poles (-21.3257, -35.5766) (-21.3578, -35.5025) (-21.4862, -35.4358) (-21.6023, -35.4358) knots 0 0 0 1 2 2 2
  spline S168 degree 2 poles (-21.6023, -35.4358) (-21.6887, -35.4358) (-21.8592, -35.5173) (-21.9382, -35.5741) knots 0 0 0 1 2 2 2
  line L224 (-21.9382, -35.5741) -> (-21.9382, -37.2019)
  line L225 (-21.9382, -37.2019) -> (-22.6545, -37.2019)
  line L226 (-22.6545, -37.2019) -> (-22.6545, -34.9023)
  line L227 (-22.6545, -34.9023) -> (-21.9382, -34.9023)
  line L228 (-21.9382, -34.9023) -> (-21.9382, -35.1567)
  spline S169 degree 2 poles (-21.9382, -35.1567) (-21.7628, -35.0085) (-21.4492, -34.8405) (-21.254, -34.8405) knots 0 0 0 1 2 2 2
  spline S170 degree 2 poles (-21.254, -34.8405) (-21.0441, -34.8405) (-20.723, -35.0406) (-20.639, -35.2407) knots 0 0 0 1 2 2 2
  spline S171 degree 2 poles (-20.639, -35.2407) (-20.434, -35.048) (-20.0684, -34.8405) (-19.8807, -34.8405) knots 0 0 0 1 2 2 2
  spline S172 degree 2 poles (-19.8807, -34.8405) (-19.7201, -34.8405) (-19.4657, -34.9418) (-19.3793, -35.0455) knots 0 0 0 1 2 2 2
  spline S173 degree 2 poles (-19.3793, -35.0455) (-19.283, -35.1567) (-19.1866, -35.4605) (-19.1866, -35.705) knots 0 0 0 1 2 2 2
  line L229 (-19.1866, -35.705) -> (-19.1866, -37.2019)
  line L230 (-19.1866, -37.2019) -> (-19.9079, -37.2019)
  spline S174 degree 2 poles (-5.1662, -36.1645) (-5.1662, -36.6461) (-5.7763, -37.2661) (-6.3098, -37.2661) knots 0 0 0 1 2 2 2
  spline S175 degree 2 poles (-6.3098, -37.2661) (-6.5765, -37.2661) (-6.994, -37.1129) (-7.1397, -36.9623) knots 0 0 0 1 2 2 2
  spline S176 degree 2 poles (-7.1397, -36.9623) (-7.3126, -36.7869) (-7.4979, -36.2312) (-7.4979, -35.8434) knots 0 0 0 1 2 2 2
  spline S177 degree 2 poles (-7.4979, -35.8434) (-7.4979, -35.4432) (-7.325, -34.8208) (-7.1298, -34.5812) knots 0 0 0 1 2 2 2
  spline S178 degree 2 poles (-7.1298, -34.5812) (-6.9446, -34.3539) (-6.3419, -34.0971) (-5.9294, -34.0971) knots 0 0 0 1 2 2 2
  spline S179 degree 2 poles (-5.9294, -34.0971) (-5.7787, -34.0971) (-5.4774, -34.1366) (-5.423, -34.1489) knots 0 0 0 1 2 2 2
  line L231 (-5.423, -34.1489) -> (-5.423, -34.7467)
  line L232 (-5.423, -34.7467) -> (-5.4774, -34.7467)
  spline S180 degree 2 poles (-5.4774, -34.7467) (-5.5317, -34.7195) (-5.7787, -34.6528) (-5.9368, -34.6528) knots 0 0 0 1 2 2 2
  spline S181 degree 2 poles (-5.9368, -34.6528) (-6.295, -34.6528) (-6.6852, -35.0307) (-6.7322, -35.3815) knots 0 0 0 1 2 2 2
  spline S182 degree 2 poles (-6.7322, -35.3815) (-6.5815, -35.2851) (-6.2727, -35.1715) (-6.0776, -35.1715) knots 0 0 0 1 2 2 2
  spline S183 degree 2 poles (-6.0776, -35.1715) (-5.9121, -35.1715) (-5.6231, -35.2604) (-5.512, -35.3444) knots 0 0 0 1 2 2 2
  spline S184 degree 2 poles (-5.512, -35.3444) (-5.3539, -35.4654) (-5.1662, -35.8582) (-5.1662, -36.1645) knots 0 0 0 1 2 2 2
  spline S185 degree 2 poles (-6.0578, -36.6239) (-5.9986, -36.5498) (-5.9343, -36.3769) (-5.9343, -36.2015) knots 0 0 0 1 2 2 2
  spline S186 degree 2 poles (-5.9343, -36.2015) (-5.9343, -36.0533) (-6.0084, -35.8606) (-6.0751, -35.8038) knots 0 0 0 1 2 2 2
  spline S187 degree 2 poles (-6.0751, -35.8038) (-6.1443, -35.7446) (-6.3147, -35.7026) (-6.4111, -35.7026) knots 0 0 0 1 2 2 2
  spline S188 degree 2 poles (-6.4111, -35.7026) (-6.4926, -35.7026) (-6.6605, -35.7446) (-6.7346, -35.7742) knots 0 0 0 1 2 2 2
  spline S189 degree 2 poles (-6.7346, -35.7742) (-6.7346, -35.794) (-6.7396, -35.8878) (-6.7396, -35.9594) knots 0 0 0 1 2 2 2
  spline S190 degree 2 poles (-6.7396, -35.9594) (-6.7396, -36.2237) (-6.6482, -36.5424) (-6.5765, -36.6239) knots 0 0 0 1 2 2 2
  spline S191 degree 2 poles (-6.5765, -36.6239) (-6.5247, -36.6906) (-6.3864, -36.7474) (-6.3122, -36.7474) knots 0 0 0 1 2 2 2
  spline S192 degree 2 poles (-6.3122, -36.7474) (-6.2505, -36.7474) (-6.1072, -36.6856) (-6.0578, -36.6239) knots 0 0 0 1 2 2 2
  line L233 (-0.7819, -37.2019) -> (-0.7819, -36.0533)
  spline S193 degree 2 poles (-0.7819, -36.0533) (-0.7819, -35.8829) (-0.7942, -35.6507) (-0.8239, -35.5766) knots 0 0 0 1 2 2 2
  spline S194 degree 2 poles (-0.8239, -35.5766) (-0.856, -35.5025) (-0.9844, -35.4358) (-1.1005, -35.4358) knots 0 0 0 1 2 2 2
  spline S195 degree 2 poles (-1.1005, -35.4358) (-1.182, -35.4358) (-1.3401, -35.5074) (-1.434, -35.5741) knots 0 0 0 1 2 2 2
  line L234 (-1.434, -35.5741) -> (-1.434, -37.2019)
  line L235 (-1.434, -37.2019) -> (-2.1552, -37.2019)
  line L236 (-2.1552, -37.2019) -> (-2.1552, -36.0533)
  spline S196 degree 2 poles (-2.1552, -36.0533) (-2.1552, -35.8853) (-2.17, -35.6507) (-2.1997, -35.5766) knots 0 0 0 1 2 2 2
  spline S197 degree 2 poles (-2.1997, -35.5766) (-2.2318, -35.5025) (-2.3602, -35.4358) (-2.4763, -35.4358) knots 0 0 0 1 2 2 2
  spline S198 degree 2 poles (-2.4763, -35.4358) (-2.5628, -35.4358) (-2.7332, -35.5173) (-2.8122, -35.5741) knots 0 0 0 1 2 2 2
  line L237 (-2.8122, -35.5741) -> (-2.8122, -37.2019)
  line L238 (-2.8122, -37.2019) -> (-3.5285, -37.2019)
  line L239 (-3.5285, -37.2019) -> (-3.5285, -34.9023)
  line L240 (-3.5285, -34.9023) -> (-2.8122, -34.9023)
  line L241 (-2.8122, -34.9023) -> (-2.8122, -35.1567)
  spline S199 degree 2 poles (-2.8122, -35.1567) (-2.6369, -35.0085) (-2.3232, -34.8405) (-2.128, -34.8405) knots 0 0 0 1 2 2 2
  spline S200 degree 2 poles (-2.128, -34.8405) (-1.9181, -34.8405) (-1.597, -35.0406) (-1.513, -35.2407) knots 0 0 0 1 2 2 2
  spline S201 degree 2 poles (-1.513, -35.2407) (-1.308, -35.048) (-0.9424, -34.8405) (-0.7547, -34.8405) knots 0 0 0 1 2 2 2
  spline S202 degree 2 poles (-0.7547, -34.8405) (-0.5942, -34.8405) (-0.3398, -34.9418) (-0.2533, -35.0455) knots 0 0 0 1 2 2 2
  spline S203 degree 2 poles (-0.2533, -35.0455) (-0.157, -35.1567) (-0.0606, -35.4605) (-0.0606, -35.705) knots 0 0 0 1 2 2 2
  line L242 (-0.0606, -35.705) -> (-0.0606, -37.2019)
  line L243 (-0.0606, -37.2019) -> (-0.7819, -37.2019)
  line L244 (3.2146, -37.2019) -> (3.2146, -36.0533)
  spline S204 degree 2 poles (3.2146, -36.0533) (3.2146, -35.8829) (3.2023, -35.6507) (3.1726, -35.5766) knots 0 0 0 1 2 2 2
  spline S205 degree 2 poles (3.1726, -35.5766) (3.1405, -35.5025) (3.0121, -35.4358) (2.896, -35.4358) knots 0 0 0 1 2 2 2
  spline S206 degree 2 poles (2.896, -35.4358) (2.8145, -35.4358) (2.6564, -35.5074) (2.5625, -35.5741) knots 0 0 0 1 2 2 2
  line L245 (2.5625, -35.5741) -> (2.5625, -37.2019)
  line L246 (2.5625, -37.2019) -> (1.8413, -37.2019)
  line L247 (1.8413, -37.2019) -> (1.8413, -36.0533)
  spline S207 degree 2 poles (1.8413, -36.0533) (1.8413, -35.8853) (1.8265, -35.6507) (1.7968, -35.5766) knots 0 0 0 1 2 2 2
  spline S208 degree 2 poles (1.7968, -35.5766) (1.7647, -35.5025) (1.6363, -35.4358) (1.5202, -35.4358) knots 0 0 0 1 2 2 2
  spline S209 degree 2 poles (1.5202, -35.4358) (1.4337, -35.4358) (1.2633, -35.5173) (1.1842, -35.5741) knots 0 0 0 1 2 2 2
  line L248 (1.1842, -35.5741) -> (1.1842, -37.2019)
  line L249 (1.1842, -37.2019) -> (0.4679, -37.2019)
  line L250 (0.4679, -37.2019) -> (0.4679, -34.9023)
  line L251 (0.4679, -34.9023) -> (1.1842, -34.9023)
  line L252 (1.1842, -34.9023) -> (1.1842, -35.1567)
  spline S210 degree 2 poles (1.1842, -35.1567) (1.3596, -35.0085) (1.6733, -34.8405) (1.8684, -34.8405) knots 0 0 0 1 2 2 2
  spline S211 degree 2 poles (1.8684, -34.8405) (2.0784, -34.8405) (2.3995, -35.0406) (2.4835, -35.2407) knots 0 0 0 1 2 2 2
  spline S212 degree 2 poles (2.4835, -35.2407) (2.6885, -35.048) (3.0541, -34.8405) (3.2418, -34.8405) knots 0 0 0 1 2 2 2
  spline S213 degree 2 poles (3.2418, -34.8405) (3.4023, -34.8405) (3.6567, -34.9418) (3.7432, -35.0455) knots 0 0 0 1 2 2 2
  spline S214 degree 2 poles (3.7432, -35.0455) (3.8395, -35.1567) (3.9358, -35.4605) (3.9358, -35.705) knots 0 0 0 1 2 2 2
  line L253 (3.9358, -35.705) -> (3.9358, -37.2019)
  line L254 (3.9358, -37.2019) -> (3.2146, -37.2019)
  line L255 (18.7959, -34.759) -> (17.4942, -37.2019)
  line L256 (17.4942, -37.2019) -> (16.6445, -37.2019)
  line L257 (16.6445, -37.2019) -> (18.0055, -34.7294)
  line L258 (18.0055, -34.7294) -> (16.5531, -34.7294)
  line L259 (16.5531, -34.7294) -> (16.5531, -34.1539)
  line L260 (16.5531, -34.1539) -> (18.7959, -34.1539)
  line L261 (18.7959, -34.1539) -> (18.7959, -34.759)
  line L262 (23.2296, -37.2019) -> (23.2296, -36.0533)
  spline S215 degree 2 poles (23.2296, -36.0533) (23.2296, -35.8829) (23.2172, -35.6507) (23.1876, -35.5766) knots 0 0 0 1 2 2 2
  spline S216 degree 2 poles (23.1876, -35.5766) (23.1555, -35.5025) (23.027, -35.4358) (22.911, -35.4358) knots 0 0 0 1 2 2 2
  spline S217 degree 2 poles (22.911, -35.4358) (22.8294, -35.4358) (22.6714, -35.5074) (22.5775, -35.5741) knots 0 0 0 1 2 2 2
  line L263 (22.5775, -35.5741) -> (22.5775, -37.2019)
  line L264 (22.5775, -37.2019) -> (21.8563, -37.2019)
  line L265 (21.8563, -37.2019) -> (21.8563, -36.0533)
  spline S218 degree 2 poles (21.8563, -36.0533) (21.8563, -35.8853) (21.8414, -35.6507) (21.8118, -35.5766) knots 0 0 0 1 2 2 2
  spline S219 degree 2 poles (21.8118, -35.5766) (21.7797, -35.5025) (21.6512, -35.4358) (21.5352, -35.4358) knots 0 0 0 1 2 2 2
  spline S220 degree 2 poles (21.5352, -35.4358) (21.4487, -35.4358) (21.2783, -35.5173) (21.1992, -35.5741) knots 0 0 0 1 2 2 2
  line L266 (21.1992, -35.5741) -> (21.1992, -37.2019)
  line L267 (21.1992, -37.2019) -> (20.4829, -37.2019)
  line L268 (20.4829, -37.2019) -> (20.4829, -34.9023)
  line L269 (20.4829, -34.9023) -> (21.1992, -34.9023)
  line L270 (21.1992, -34.9023) -> (21.1992, -35.1567)
  spline S221 degree 2 poles (21.1992, -35.1567) (21.3746, -35.0085) (21.6883, -34.8405) (21.8834, -34.8405) knots 0 0 0 1 2 2 2
  spline S222 degree 2 poles (21.8834, -34.8405) (22.0934, -34.8405) (22.4145, -35.0406) (22.4985, -35.2407) knots 0 0 0 1 2 2 2
  spline S223 degree 2 poles (22.4985, -35.2407) (22.7035, -35.048) (23.069, -34.8405) (23.2568, -34.8405) knots 0 0 0 1 2 2 2
  spline S224 degree 2 poles (23.2568, -34.8405) (23.4173, -34.8405) (23.6717, -34.9418) (23.7582, -35.0455) knots 0 0 0 1 2 2 2
  spline S225 degree 2 poles (23.7582, -35.0455) (23.8545, -35.1567) (23.9508, -35.4605) (23.9508, -35.705) knots 0 0 0 1 2 2 2
  line L271 (23.9508, -35.705) -> (23.9508, -37.2019)
  line L272 (23.9508, -37.2019) -> (23.2296, -37.2019)
  line L273 (27.2261, -37.2019) -> (27.2261, -36.0533)
  spline S226 degree 2 poles (27.2261, -36.0533) (27.2261, -35.8829) (27.2137, -35.6507) (27.1841, -35.5766) knots 0 0 0 1 2 2 2
  spline S227 degree 2 poles (27.1841, -35.5766) (27.152, -35.5025) (27.0235, -35.4358) (26.9074, -35.4358) knots 0 0 0 1 2 2 2
  spline S228 degree 2 poles (26.9074, -35.4358) (26.8259, -35.4358) (26.6678, -35.5074) (26.574, -35.5741) knots 0 0 0 1 2 2 2
  line L274 (26.574, -35.5741) -> (26.574, -37.2019)
  line L275 (26.574, -37.2019) -> (25.8527, -37.2019)
  line L276 (25.8527, -37.2019) -> (25.8527, -36.0533)
  spline S229 degree 2 poles (25.8527, -36.0533) (25.8527, -35.8853) (25.8379, -35.6507) (25.8083, -35.5766) knots 0 0 0 1 2 2 2
  spline S230 degree 2 poles (25.8083, -35.5766) (25.7762, -35.5025) (25.6477, -35.4358) (25.5316, -35.4358) knots 0 0 0 1 2 2 2
  spline S231 degree 2 poles (25.5316, -35.4358) (25.4452, -35.4358) (25.2748, -35.5173) (25.1957, -35.5741) knots 0 0 0 1 2 2 2
  line L277 (25.1957, -35.5741) -> (25.1957, -37.2019)
  line L278 (25.1957, -37.2019) -> (24.4794, -37.2019)
  line L279 (24.4794, -37.2019) -> (24.4794, -34.9023)
  line L280 (24.4794, -34.9023) -> (25.1957, -34.9023)
  line L281 (25.1957, -34.9023) -> (25.1957, -35.1567)
  spline S232 degree 2 poles (25.1957, -35.1567) (25.3711, -35.0085) (25.6848, -34.8405) (25.8799, -34.8405) knots 0 0 0 1 2 2 2
  spline S233 degree 2 poles (25.8799, -34.8405) (26.0899, -34.8405) (26.411, -35.0406) (26.4949, -35.2407) knots 0 0 0 1 2 2 2
  spline S234 degree 2 poles (26.4949, -35.2407) (26.7, -35.048) (27.0655, -34.8405) (27.2532, -34.8405) knots 0 0 0 1 2 2 2
  spline S235 degree 2 poles (27.2532, -34.8405) (27.4138, -34.8405) (27.6682, -34.9418) (27.7547, -35.0455) knots 0 0 0 1 2 2 2
  spline S236 degree 2 poles (27.7547, -35.0455) (27.851, -35.1567) (27.9473, -35.4605) (27.9473, -35.705) knots 0 0 0 1 2 2 2
  line L282 (27.9473, -35.705) -> (27.9473, -37.2019)
  line L283 (27.9473, -37.2019) -> (27.2261, -37.2019)
  spline S237 degree 2 poles (43.7557, -36.3547) (43.7557, -36.5498) (43.5926, -36.8882) (43.437, -37.0117) knots 0 0 0 1 2 2 2
  spline S238 degree 2 poles (43.437, -37.0117) (43.2814, -37.1352) (42.8343, -37.2735) (42.5453, -37.2735) knots 0 0 0 1 2 2 2
  spline S239 degree 2 poles (42.5453, -37.2735) (42.2366, -37.2735) (41.7747, -37.1327) (41.6265, -37.0117) knots 0 0 0 1 2 2 2